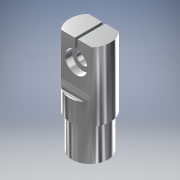
# Autodesk Inventor part: koncowka
Saved by Autodesk Inventor 2017 (Build 210142000, 142)
## iProperties
Created: 2017-03-22
Part Number: koncowka
Material: Aluminium 6061
Document SubType Name: Modeling
Designer: Damian
Density: 2.7 g/cm^3
Appearance: Aluminium — płaski
Mass: 109.909 g
Surface Area: 93.9656 cm^2
Volume: 40.7069 cm^3
Author: Damian
Autodesk Inventor part; units mm, degrees
ref_plane "YZ Plane" through (0, 0, 0) normal (1, 0, 0) x (0, 1, 0)
ref_plane "XZ Plane" through (0, 0, 0) normal (0, 1, 0) x (-1, 0, 0)
ref_plane "XY Plane" through (0, 0, 0) normal (0, 0, 1) x (1, 0, 0)
sketch "Szkic1" plane through (0, 0, 0) normal (0, 0, 1) x (1, 0, 0)
  circle A0 centre (0, 0) radius 15
  dimension "d0" = 30
  constraints: 1 centre point, 1 coincident
  measures "d0" diameter of A0
extrude "Wyciągnięcie proste1" add sketch "Szkic1" along normal mid plane 75
sketch "Szkic2" plane through (0, 0, -37.5) normal (0, 0, -1) x (-1, 0, 0)
  circle A0 centre (0, 0) radius 13
  circle A1 centre (0, 0) radius 15
  dimension "d3" = 26
  dimension "d4" = 30
  constraints: 3 coincident, 2 centre point
  measures "d3" diameter of A0
  measures "d4" diameter of A1
extrude "Wyciągnięcie proste2" cut sketch "Szkic2" against normal blind 25
sketch "Szkic3" plane through (0, 0, 0) normal (1, 0, 0) x (0, 1, 0)
  circle A0 centre (0, -32.5) radius 1.5
  circle A1 centre (0, -22.5) radius 1.5
  line L0 (-13, -37.5) -> (13, -37.5) projected
  point P0 (0, 0)
  dimension "d7" = 3
  dimension "d8" = 3
  dimension "d13" = 10
  dimension "d14" = 5
  constraints: 2 centre point
  measures "d7" diameter of A0
  measures "d8" diameter of A1
  measures "d13" distance of A1.centre A0.centre
  measures "d14" distance from line of L0 A0.centre
extrude "Wyciągnięcie proste3" cut sketch "Szkic3" against normal blind 25 and the other way blind 12.5
thread "Gwint1" size "M3x0.5" class "6H" standard "ANSI Metric M Profile" full length
thread "Gwint2" size "M3x0.5" class "6H" standard "ANSI Metric M Profile" full length
sketch "Szkic4" plane through (0, 0, 0) normal (1, 0, 0) x (0, 1, 0)
  line L0 (15, 37.5) -> (-15, 37.5) projected
  line L1 (-15, 37.5) -> (-10, 37.5)
  line L2 (-10, 37.5) -> (-10, 7.5)
  line L3 (-15, 2.5) -> (-15, 2.5)
  line L4 (-15, 2.5) -> (-15, 37.5)
  line L5 (15, 37.5) -> (10, 37.5)
  line L6 (10, 37.5) -> (10, 7.5)
  line L7 (15, 2.5) -> (15, 2.5)
  line L8 (15, 2.5) -> (15, 37.5)
  arc A0 (-15, 2.5) -> (-10, 7.5) centre (-15, 7.5) ccw
  arc A1 (10, 7.5) -> (15, 2.5) centre (15, 7.5) ccw
  point P0 (0, 0)
  point P1 (-10, 2.5)
  point P2 (10, 2.5)
  dimension "d19" = 5
  dimension "d20" = 35
  dimension "d21" = 5
  dimension "d22" = 35
  dimension "d25" = 5
  dimension "d26" = 5
  constraints: 16 end point, 4 parallel, 4 point on circle, 4 point on line, 4 tangent, 2 centre point, 2 horizontal, 2 perpendicular
  measures "d19" distance of point (-10, 2.5) L3.end
  measures "d20" distance of L1.end point (-10, 2.5)
  measures "d21" distance of L7.end point (10, 2.5)
  measures "d22" distance of point (10, 2.5) L5.end
  measures "d25" radius of A0
  measures "d26" radius of A1
extrude "Wyciągnięcie proste4" cut sketch "Szkic4" along normal mid plane 30
sketch "Szkic6" plane through (-11.1803, 10, 7.5) normal (0, 1, 0) x (1, 0, 0)
  line L0 (-3.8197, -30) -> (0, -30) construction
  line L1 (0, 0) -> (22.3607, 0) construction
  line L2 (0, -30) -> (22.3607, -30) construction
  line L3 (22.3607, -30) -> (22.3607, 0) construction
  line L4 (22.3607, 0) -> (0, 0) construction
  line L5 (0, 0) -> (0, -30) construction
  circle A0 centre (11.1803, -15) radius 8.05
  point P0 (11.1803, 7.5)
  dimension "d30" = 16.1
  constraints: 8 end point, 2 parallel, 1 centre point, 1 horizontal, 1 perpendicular
  measures "d30" diameter of A0
extrude "Wyciągnięcie proste6" cut sketch "Szkic6" against normal blind 5
sketch "Szkic7" plane through (0, 5, 22.5) normal (0, 1, 0) x (1, 0, 0)
  circle A0 centre (0, 0) radius 4.5
  point P0 (0, 22.5)
  dimension "d33" = 9
  constraints: 1 centre point
  measures "d33" diameter of A0
extrude "Wyciągnięcie proste7" cut sketch "Szkic7" against normal blind 30
sketch "Szkic8" plane through (0, 0, 37.5) normal (0, 0, 1) x (1, 0, 0)
  line L0 (-1, 10) -> (1, 10)
  line L1 (1, 10) -> (1, -10)
  line L2 (1, -10) -> (-1, -10)
  line L3 (-1, -10) -> (-1, 10)
  line L4 (-1, 10) -> (1, -10) construction
  line L5 (1, 10) -> (-1, -10) construction
  point P0 (0, 0)
  dimension "d36" = 2
  dimension "d37" = 20
  constraints: 12 end point, 2 midpoint, 2 parallel, 1 horizontal, 1 perpendicular
  measures "d36" distance of L1.end L2.end
  measures "d37" distance of L0.end L1.end
extrude "Wyciągnięcie proste8" cut sketch "Szkic8" against normal blind 12
sketch "Szkic9" plane through (1, -10, 37.5) normal (-1, 0, 0) x (0, 0, 1)
  circle A0 centre (-3.5, 10) radius 1.5
  point P0 (-37.5, 10)
  dimension "d40" = 3
  constraints: 1 centre point
  measures "d40" diameter of A0
extrude "Wyciągnięcie proste9" cut sketch "Szkic9" against normal blind 10 and the other way blind 20
thread "Gwint3" size "M3x0.5" class "6H" standard "ANSI Metric M Profile" full length
sketch "Szkic10" plane through (-11.1803, -10, 7.5) normal (0, -1, 0) x (1, 0, 0)
  arc A0 (10.1803, 19.3875) -> (12.1803, 19.3875) centre (11.1803, 15) ccw projected
  circle A1 centre (11.1803, 15) radius 8.05
  point P0 (11.1803, -7.5)
  dimension "d49" = 16.1
  constraints: 1 centre point, 1 coincident
  measures "d49" diameter of A1
extrude "Wyciągnięcie proste10" cut sketch "Szkic10" against normal blind 5
chamfer "Faza1" distance 2 angle 45 1 edges at (-15, -0.0202, 32.5001)
equation "\"d21\" = d19"
equation "\"d22\" = d20"
equation "\"d26\" = d25"
